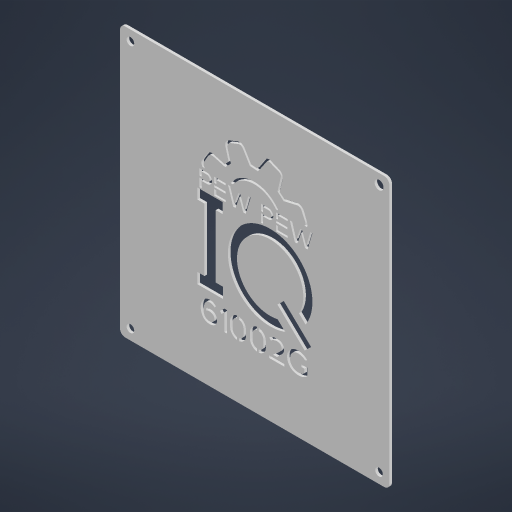
# Autodesk Inventor part: cutout
Saved by Autodesk Inventor 2024 (Build 280153000, 153)
## iProperties
Created: 2023-09-04
Part Number: cutout
Material: Generic
Document SubType Name: Modeling
Designer: reima
Density: 1 g/cm^3
Appearance: Default
Author: reima
Autodesk Inventor part; units mm, degrees
ref_plane "YZ Plane" through (0, 0, 0) normal (1, 0, 0) x (0, 1, 0)
ref_plane "XZ Plane" through (0, 0, 0) normal (0, 1, 0) x (-1, 0, 0)
ref_plane "XY Plane" through (0, 0, 0) normal (0, 0, 1) x (1, 0, 0)
sketch "Sketch1" plane through (0, 0, 0) normal (0, 0, 1) x (1, 0, 0)
  line L0 (-79.375, 82.55) -> (79.375, 82.55)
  line L1 (82.55, 79.375) -> (82.55, -79.375)
  line L2 (79.375, -82.55) -> (-79.375, -82.55)
  line L3 (-82.55, -79.375) -> (-82.55, 79.375)
  arc A0 (-79.375, 82.55) -> (-82.55, 79.375) centre (-79.375, 79.375) ccw
  arc A1 (-82.55, -79.375) -> (-79.375, -82.55) centre (-79.375, -79.375) ccw
  arc A2 (79.375, -82.55) -> (82.55, -79.375) centre (79.375, -79.375) ccw
  arc A3 (82.55, 79.375) -> (79.375, 82.55) centre (79.375, 79.375) ccw
  circle A4 centre (-76.2, 76.2) radius 2.3368
  circle A5 centre (76.2, 76.2) radius 2.7491
  circle A6 centre (76.2, -76.2) radius 2.3368
  circle A7 centre (-76.2, -76.2) radius 2.3368
  point P0 (0, 0)
  point P1 (-82.55, 82.55)
  point P2 (82.55, -82.55)
  point P3 (82.55, 82.55)
  dimension "d0" = 165.1
  dimension "d1" = 165.1
  dimension "d2" = 3.175
  dimension "d3" = 4.6736
  dimension "d4" = 6.35
  dimension "d5" = 6.35
  dimension "d6" = 4.6736
  dimension "d7" = 6.35
  dimension "d8" = 6.35
  dimension "d9" = 6.35
  dimension "d10" = 6.35
  dimension "d11" = 4.6736
  dimension "d12" = 6.35
  dimension "d13" = 6.35
  dimension "d16" = 82.55
  dimension "d17" = 82.55
  constraints: 8 centre point, 8 end point, 8 point on circle, 8 tangent, 6 point on line, 3 equal radius, 2 parallel, 1 horizontal, 1 perpendicular
  measures "d0" distance of point (-82.55, 82.55) point (82.55, 82.55)
  measures "d1" distance of point (82.55, 82.55) point (82.55, -82.55)
  measures "d2" radius of A0
  measures "d3" diameter of A4
  measures "d4" distance from line of L0 A4.centre
  measures "d5" distance from line of L3 A4.centre
  measures "d6" diameter of A7
  measures "d7" distance from line of L3 A7.centre
  measures "d8" distance from line of L2 A7.centre
  measures "d9" distance from line of L0 A5.centre
  measures "d10" distance from line of L1 A5.centre
  measures "d11" diameter of A6
  measures "d12" distance from line of L1 A6.centre
  measures "d13" distance from line of L2 A6.centre
  measures "d16" distance from line of point (0, 0) L0
  measures "d17" distance from line of point (0, 0) L3
extrude "Extrusion1" add sketch "Sketch1" along normal blind 1.5875
sketch "Sketch2" plane through (0, 0, 1.5875) normal (0, 0, 1) x (1, 0, 0)
  line L0 (79.375, 82.55) -> (-79.375, 82.55) projected
  line L1 (-82.55, 79.375) -> (-82.55, -79.375) projected
  line L2 (82.55, -79.375) -> (82.55, 79.375) projected
  line L3 (-79.375, -82.55) -> (79.375, -82.55) projected
  line L4 (-24.8519, 25.6674) -> (-17.8481, 25.6674)
  line L5 (-17.8481, 25.6674) -> (-17.8481, 24.5342)
  line L6 (-17.8481, 24.5342) -> (-24.8519, 24.5342)
  line L7 (-24.8519, 24.5342) -> (-24.8519, 25.6674)
  line L8 (-24.8519, 23.4797) -> (-23.5456, 23.4797)
  line L9 (-23.5456, 23.4797) -> (-23.5456, 20.0486)
  line L10 (-23.5456, 20.0486) -> (-24.8519, 20.0486)
  line L11 (-24.8519, 20.0486) -> (-24.8519, 23.4797)
  line L12 (-23.5456, 20.0486) -> (-17.8481, 20.0486)
  line L13 (-17.8481, 20.0486) -> (-17.8481, 21.1661)
  line L14 (-17.8481, 21.1661) -> (-23.5456, 21.1661)
  line L15 (-23.5456, 21.1661) -> (-23.5456, 20.0486)
  line L16 (-24.8519, 26.8478) -> (-23.5456, 26.8478)
  line L17 (-23.5456, 26.8478) -> (-23.5456, 30.0743)
  line L18 (-23.5456, 30.0743) -> (-24.8519, 30.0743)
  line L19 (-24.8519, 30.0743) -> (-24.8519, 26.8478)
  line L20 (-23.5456, 30.0743) -> (-17.8481, 30.0743)
  line L21 (-17.8481, 30.0743) -> (-17.8481, 28.9568)
  line L22 (-17.8481, 28.9568) -> (-23.5456, 28.9568)
  line L23 (-23.5456, 28.9568) -> (-23.5456, 30.0743)
  line L24 (-33.9115, 26.22) -> (-32.605, 26.22)
  line L25 (-32.605, 26.22) -> (-32.605, 30.0743)
  line L26 (-32.605, 30.0743) -> (-33.9115, 30.0743)
  line L27 (-33.9115, 30.0743) -> (-33.9115, 26.22)
  line L28 (-33.9115, 25.1008) -> (-32.605, 25.1008)
  line L29 (-32.605, 25.1008) -> (-32.605, 20.0486)
  line L30 (-32.605, 20.0486) -> (-33.9115, 20.0486)
  line L31 (-33.9115, 20.0486) -> (-33.9115, 25.1008)
  line L32 (-32.605, 30.0743) -> (-29.4768, 30.0743)
  line L33 (-29.4768, 30.0743) -> (-29.4768, 28.9568)
  line L34 (-29.4768, 28.9568) -> (-32.605, 28.9568)
  line L35 (-32.605, 28.9568) -> (-32.605, 30.0743)
  line L36 (-32.605, 25.1008) -> (-29.4768, 25.1008)
  line L37 (-29.4768, 25.1008) -> (-29.4768, 24.0088)
  line L38 (-29.4768, 24.0088) -> (-32.605, 24.0088)
  line L39 (-32.605, 24.0088) -> (-32.605, 25.1008)
  arc A0 (-29.4768, 25.1008) -> (-29.4768, 28.9568) centre (-29.4768, 27.0288) ccw
  arc A1 (-29.4768, 24.0088) -> (-29.4768, 30.0743) centre (-29.2319, 27.0416) ccw
  line L40 (-16.4079, 30.0743) -> (-15.0487, 30.0064)
  line L41 (-15.0487, 30.0064) -> (-12.5084, 21.995)
  line L42 (-12.5084, 21.995) -> (-9.9795, 28.8267)
  line L43 (-9.9795, 28.8267) -> (-8.8388, 28.8267)
  line L44 (-8.8388, 28.8267) -> (-6.3295, 21.6605)
  line L45 (-6.3295, 21.6605) -> (-3.9885, 30.0743)
  line L46 (-3.9885, 30.0743) -> (-2.5145, 30.0743)
  line L47 (-2.5145, 30.0743) -> (-5.4869, 20.0486)
  line L48 (-5.4869, 20.0486) -> (-7.0427, 20.0486)
  line L49 (-7.0427, 20.0486) -> (-9.4296, 26.8478)
  line L50 (-9.4296, 26.8478) -> (-11.7613, 20.0486)
  line L51 (-11.7613, 20.0486) -> (-13.2289, 20.0486)
  line L52 (-16.4079, 30.0743) -> (-13.2289, 20.0486)
  line L53 (3.7905, 26.22) -> (5.0925, 26.22)
  line L54 (5.0925, 26.22) -> (5.0925, 30.0743)
  line L55 (5.0925, 30.0743) -> (3.7905, 30.0743)
  line L56 (3.7905, 30.0743) -> (3.7905, 26.22)
  line L57 (3.7905, 25.0615) -> (5.0925, 25.0615)
  line L58 (5.0925, 25.0615) -> (5.0925, 20.0486)
  line L59 (5.0925, 20.0486) -> (3.7905, 20.0486)
  line L60 (3.7905, 20.0486) -> (3.7905, 25.0615)
  line L61 (5.0925, 30.0743) -> (8.1235, 30.0743)
  line L62 (8.1235, 30.0743) -> (8.1235, 28.9568)
  line L63 (8.1235, 28.9568) -> (5.0925, 28.9568)
  line L64 (5.0925, 28.9568) -> (5.0925, 30.0743)
  line L65 (5.0925, 25.0615) -> (8.1235, 25.0615)
  line L66 (8.1235, 25.0615) -> (8.1235, 24.0088)
  line L67 (8.1235, 24.0088) -> (5.0925, 24.0088)
  line L68 (5.0925, 24.0088) -> (5.0925, 25.0615)
  arc A2 (8.1235, 25.0615) -> (8.1235, 28.9568) centre (8.2489, 27.0091) ccw
  arc A3 (8.1235, 24.0088) -> (8.1235, 30.0743) centre (8.318, 27.0416) ccw
  line L69 (12.9709, 30.0743) -> (20.1584, 30.0743)
  line L70 (20.1584, 30.0743) -> (20.1584, 28.9568)
  line L71 (20.1584, 28.9568) -> (12.9709, 28.9568)
  line L72 (12.9709, 28.9568) -> (12.9709, 30.0743)
  line L73 (12.9709, 30.0743) -> (14.2728, 30.0743)
  line L74 (14.2728, 30.0743) -> (14.2728, 26.8478)
  line L75 (14.2728, 26.8478) -> (12.9709, 26.8478)
  line L76 (12.9709, 26.8478) -> (12.9709, 30.0743)
  line L77 (12.9709, 25.6674) -> (19.9716, 25.6674)
  line L78 (19.9716, 25.6674) -> (19.9716, 24.5352)
  line L79 (19.9716, 24.5352) -> (12.9709, 24.5352)
  line L80 (12.9709, 24.5352) -> (12.9709, 25.6674)
  line L81 (12.9709, 23.4482) -> (14.2728, 23.4482)
  line L82 (14.2728, 23.4482) -> (14.2728, 20.0486)
  line L83 (14.2728, 20.0486) -> (12.9709, 20.0486)
  line L84 (12.9709, 20.0486) -> (12.9709, 23.4482)
  line L85 (14.2728, 20.0486) -> (20.1584, 20.0486)
  line L86 (20.1584, 20.0486) -> (20.1584, 21.1661)
  line L87 (20.1584, 21.1661) -> (14.2728, 21.1661)
  line L88 (14.2728, 21.1661) -> (14.2728, 20.0486)
  line L89 (21.5158, 30.0743) -> (22.9913, 30.0743)
  line L90 (22.9913, 30.0743) -> (25.3697, 21.9057)
  line L91 (25.3697, 21.9057) -> (27.9414, 28.8267)
  line L92 (27.9414, 28.8267) -> (29.0321, 28.8267)
  line L93 (29.0321, 28.8267) -> (31.5461, 21.6605)
  line L94 (31.5461, 21.6605) -> (34.0406, 30.0743)
  line L95 (34.0406, 30.0743) -> (35.364, 30.0743)
  line L96 (35.364, 30.0743) -> (32.3916, 20.0486)
  line L97 (32.3916, 20.0486) -> (30.821, 20.0486)
  line L98 (30.821, 20.0486) -> (28.4867, 26.9432)
  line L99 (28.4867, 26.9432) -> (26.1223, 20.0486)
  line L100 (26.1223, 20.0486) -> (24.5757, 20.0486)
  line L101 (24.5757, 20.0486) -> (21.5158, 30.0743)
  line L102 (-14.8184, 31.7504) -> (-13.3796, 31.7504)
  line L103 (14.4691, 31.7504) -> (12.9504, 31.7504)
  arc A4 (12.9504, 31.7504) -> (-13.3796, 31.7504) centre (-0.2146, 22.0306) ccw
  arc A5 (14.4691, 31.7504) -> (-14.8184, 31.7504) centre (-0.1747, 22.2165) ccw
  arc A6 (-30.8376, 35.2446) -> (-30.528, 31.7301) centre (-28.5658, 33.6739) ccw
  arc A7 (-24.9796, 40.4718) -> (-28.5658, 39.1347) centre (-25.9768, 37.6683) ccw
  arc A8 (-7.2899, 53.8438) -> (-10.3551, 54.6808) centre (-9.252, 52.6894) ccw
  arc A9 (9.174, 54.763) -> (7.322, 54.1112) centre (8.6906, 53.1796) ccw
  arc A10 (15.9892, 50.348) -> (15.2336, 52.3036) centre (14.2988, 50.8186) ccw
  arc A11 (30.4954, 31.7302) -> (30.6342, 34.6691) centre (28.6879, 33.2883) ccw
  arc A12 (28.7936, 38.6923) -> (26.0478, 40.3102) centre (26.5711, 38.0594) ccw
  line L104 (17.7398, 38.395) -> (26.0478, 40.3102)
  line L105 (28.7936, 38.6923) -> (30.6342, 34.6691)
  line L106 (30.4954, 31.7302) -> (31.9789, 31.7302)
  line L107 (-7.2899, 53.8438) -> (-2.9717, 46.7093)
  line L108 (-2.9717, 46.7093) -> (2.0382, 46.3701)
  line L109 (2.0382, 46.3701) -> (7.322, 54.1112)
  line L110 (9.174, 54.763) -> (15.2336, 52.3036)
  line L111 (15.9892, 50.348) -> (13.9731, 41.6604)
  line L112 (13.9731, 41.6604) -> (17.7398, 38.395)
  line L113 (-30.8376, 35.2446) -> (-28.5658, 39.1347)
  line L114 (-24.9796, 40.4718) -> (-18.0625, 38.5471)
  line L115 (-18.0625, 38.5471) -> (-14.6127, 42.0733)
  line L116 (-14.6127, 42.0733) -> (-16.6084, 49.3312)
  line L117 (-30.528, 31.7301) -> (-32.0036, 31.7301)
  arc A13 (-32.3999, 35.0685) -> (-32.0036, 31.7301) centre (-29.3965, 33.7324) ccw
  arc A14 (-25.3886, 41.886) -> (-27.8196, 41.5513) centre (-26.1227, 38.2222) ccw
  line L118 (-32.3999, 35.0685) -> (-28.8099, 40.8187)
  arc A15 (-27.8196, 41.5513) -> (-28.8099, 40.8187) centre (-26.1228, 38.2221) ccw
  line L119 (-25.3886, 41.886) -> (-18.5094, 39.8807)
  line L120 (-18.5094, 39.8807) -> (-15.9824, 42.4637)
  line L121 (-15.9824, 42.4637) -> (-17.782, 49.0085)
  arc A16 (-15.4658, 52.6898) -> (-16.6084, 49.3312) centre (-13.5626, 50.1687) ccw
  line L122 (-15.4658, 52.6898) -> (-10.3551, 54.6808)
  arc A17 (-16.0392, 53.8438) -> (-17.9814, 49.7337) centre (-14.5412, 50.622) ccw
  line L123 (-17.9814, 49.7337) -> (-17.782, 49.0085)
  arc A18 (-6.1258, 54.5484) -> (-10.1949, 56.0828) centre (-9.119, 52.7734) ccw
  line L124 (-16.0392, 53.8438) -> (-10.1949, 56.0828)
  line L125 (-6.1258, 54.5484) -> (-2.1918, 47.9531)
  line L126 (-2.1918, 47.9531) -> (1.4246, 47.6353)
  arc A19 (10.2006, 55.7927) -> (6.1245, 54.7631) centre (8.8209, 52.6717) ccw
  line L127 (1.4246, 47.6353) -> (6.1245, 54.7631)
  arc A20 (17.0893, 49.5812) -> (15.5262, 53.5334) centre (13.7637, 50.5511) ccw
  line L128 (17.0893, 49.5812) -> (15.3353, 42.0229)
  line L129 (10.2006, 55.7927) -> (15.5262, 53.5334)
  line L130 (15.3353, 42.0229) -> (18.1443, 39.6904)
  arc A21 (30.2891, 39.005) -> (25.8497, 41.5513) centre (26.659, 37.8191) ccw
  line L131 (25.8497, 41.5513) -> (18.1443, 39.6904)
  arc A22 (31.9789, 31.7302) -> (32.1682, 34.1841) centre (29.8071, 33.132) ccw
  line L132 (30.2891, 39.005) -> (32.1682, 34.1841)
  line L133 (-35.213, 19.1945) -> (-19.5698, 19.1945)
  line L134 (-19.5698, 19.1945) -> (-19.5698, 12.8212)
  line L135 (-19.5698, 12.8212) -> (-35.213, 12.8212)
  line L136 (-35.213, 12.8212) -> (-35.213, 19.1945)
  line L137 (-30.7892, 12.8212) -> (-23.8688, 12.8212)
  line L138 (-23.8688, 12.8212) -> (-23.8688, -25.645)
  line L139 (-23.8688, -25.645) -> (-30.7892, -25.645)
  line L140 (-30.7892, -25.645) -> (-30.7892, 12.8212)
  line L141 (-35.213, -25.645) -> (-19.5138, -25.645)
  line L142 (-19.5138, -25.645) -> (-19.5138, -32.1253)
  line L143 (-19.5138, -32.1253) -> (-35.213, -32.1253)
  line L144 (-35.213, -32.1253) -> (-35.213, -25.645)
  line L145 (17.8686, -14.6278) -> (13.8767, -18.395)
  line L146 (13.8767, -18.395) -> (30.6342, -34.4875)
  line L147 (30.6342, -34.4875) -> (34.6261, -30.7203)
  line L148 (34.6261, -30.7203) -> (17.8686, -14.6278)
  arc A23 (27.1093, -16.4401) -> (14.0046, -26.1551) centre (9.4734, -6.3468) ccw
  arc A24 (31.9416, -19.2058) -> (15.2462, -31.5827) centre (9.4734, -6.3468) ccw
  line L149 (14.0046, -26.1551) -> (18.6982, -30.5352)
  arc A25 (15.2462, -31.5827) -> (18.6982, -30.5352) centre (9.4734, -6.3468) ccw
  line L150 (27.1093, -16.4401) -> (31.1956, -20.4294)
  arc A26 (31.1956, -20.4294) -> (31.949, -19.1929) centre (9.4734, -6.3468) ccw
  line L151 (-16.961, -49.284) -> (-18.6004, -49.284)
  line L152 (-18.6004, -49.284) -> (-18.6004, -36.8327)
  line L153 (-18.6004, -36.8327) -> (-16.961, -36.8327)
  line L154 (-16.961, -36.8327) -> (-16.961, -49.284)
  line L155 (-18.6004, -36.8327) -> (-21.35, -39.4034)
  line L156 (-21.35, -39.4034) -> (-20.2834, -40.5442)
  line L157 (-20.2834, -40.5442) -> (-18.6004, -38.8165)
  line L158 (8.8648, -47.9011) -> (18.2227, -47.9011)
  line L159 (18.2227, -47.9011) -> (18.2227, -49.284)
  line L160 (18.2227, -49.284) -> (8.8648, -49.284)
  line L161 (8.8648, -49.284) -> (8.8648, -47.9011)
  line L162 (28.559, -42.8648) -> (32.2489, -42.8648)
  line L163 (32.2489, -42.8648) -> (32.2489, -44.216)
  line L164 (32.2489, -44.216) -> (28.559, -44.216)
  line L165 (28.559, -44.216) -> (28.559, -42.8648)
  line L166 (-24.5421, -39.1949) -> (-23.7981, -38.118)
  arc A27 (-23.7981, -38.118) -> (-32.0782, -39.1949) centre (-27.5277, -41.8118) ccw
  arc A28 (-32.0782, -39.1949) -> (-31.5922, -47.9011) centre (-25.0317, -43.1683) ccw
  arc A29 (-31.5922, -47.9011) -> (-24.8519, -48.7501) centre (-27.7037, -44.2105) ccw
  arc A30 (-24.8519, -48.7501) -> (-23.4202, -43.7641) centre (-27.0708, -45.4145) ccw
  arc A31 (-23.4202, -43.7641) -> (-27.1885, -41.472) centre (-26.7816, -45.0466) ccw
  line L167 (-29.7906, -42.2565) -> (-29.7906, -43.2994)
  arc A32 (-25.7118, -43.4813) -> (-29.7906, -43.2994) centre (-27.9049, -46.8361) ccw
  line L168 (-27.1885, -41.472) -> (-28.3737, -41.472)
  arc A33 (-28.3737, -41.472) -> (-29.7906, -42.2565) centre (-28.4926, -42.9291) ccw
  arc A34 (-25.8864, -47.5561) -> (-25.7118, -43.4813) centre (-27.1461, -45.461) ccw
  arc A35 (-30.703, -46.5882) -> (-25.8864, -47.5561) centre (-27.8144, -44.6818) ccw
  arc A36 (-31.3171, -43.1683) -> (-30.703, -46.5882) centre (-25.48, -43.8852) ccw
  arc A37 (-30.7892, -40.3427) -> (-31.3171, -43.1683) centre (-15.1595, -44.725) ccw
  arc A38 (-26.8428, -38.0151) -> (-30.7892, -40.3427) centre (-27.433, -41.5238) ccw
  arc A39 (-24.5421, -39.1949) -> (-26.8428, -38.0151) centre (-28.5537, -44.1848) ccw
  arc A40 (-6.8639, -41.3097) -> (-13.5626, -41.3297) centre (-10.2129, -41.4212) ccw
  arc A41 (-13.5626, -44.9246) -> (-6.8639, -44.9246) centre (-10.2132, -44.7281) ccw
  line L169 (-13.5626, -41.3297) -> (-13.5626, -44.9246)
  line L170 (-6.8639, -41.3097) -> (-6.8639, -44.9246)
  arc A42 (5.2396, -41.3097) -> (-1.3131, -41.3097) centre (1.9632, -41.346) ccw
  arc A43 (-1.3131, -45.0466) -> (5.2396, -44.9246) centre (1.9597, -44.7941) ccw
  line L171 (-1.3131, -41.3097) -> (-1.3131, -45.0466)
  line L172 (5.2396, -41.3097) -> (5.2396, -44.9246)
  arc A44 (-5.3567, -41.2869) -> (-15.0698, -41.311) centre (-10.2129, -41.4212) ccw
  line L173 (-5.3567, -41.2869) -> (-5.3567, -44.9647)
  arc A45 (-15.0698, -44.9647) -> (-5.3567, -44.9647) centre (-10.2132, -44.7281) ccw
  line L174 (-15.0698, -44.9647) -> (-15.0698, -41.311)
  arc A46 (-2.9246, -45.1025) -> (6.8511, -44.9535) centre (1.9597, -44.7941) ccw
  line L175 (6.8511, -44.9535) -> (6.8511, -41.3016)
  arc A47 (6.8511, -41.3016) -> (-2.9246, -41.3016) centre (1.9632, -41.346) ccw
  line L176 (-2.9246, -41.3016) -> (-2.9246, -45.1025)
  arc A48 (14.4691, -38.0695) -> (9.9205, -39.5089) centre (13.7247, -43.6238) ccw
  arc A49 (16.0784, -38.9953) -> (14.4691, -38.0695) centre (13.7834, -41.1229) ccw
  arc A50 (16.2123, -41.472) -> (16.0784, -38.9953) centre (13.9632, -40.3516) ccw
  arc A51 (13.8767, -44.1033) -> (16.2123, -41.472) centre (8.8032, -37.2477) ccw
  line L177 (11.1363, -46.3974) -> (13.8767, -44.1033)
  line L178 (11.1363, -46.3974) -> (13.6219, -46.3974)
  line L179 (13.6219, -46.3974) -> (16.0784, -44.1033)
  arc A52 (16.0784, -44.1033) -> (17.6164, -42.0514) centre (10.1369, -38.0474) ccw
  arc A53 (17.6164, -42.0514) -> (17.7841, -38.8995) centre (14.3385, -40.2966) ccw
  arc A54 (17.7679, -38.8601) -> (14.911, -36.7775) centre (14.5315, -40.2988) ccw
  line L180 (17.7679, -38.8601) -> (17.7841, -38.8995)
  arc A55 (14.911, -36.7775) -> (11.4325, -36.9516) centre (13.7088, -47.5948) ccw
  arc A56 (11.4325, -36.9516) -> (8.8648, -38.4103) centre (12.8598, -42.4531) ccw
  line L181 (8.8648, -38.4103) -> (9.9205, -39.5089)
  line L182 (-9.5656, -36.6064) -> (-10.8602, -36.6064)
  line L183 (-10.8602, -36.6064) -> (-10.8602, -49.6876)
  line L184 (-10.8602, -49.6876) -> (-9.5656, -49.6876)
  line L185 (-9.5656, -49.6876) -> (-9.5656, -36.6064)
  line L186 (1.4246, -36.4878) -> (2.5019, -36.4878)
  line L187 (2.5019, -36.4878) -> (2.5019, -49.6876)
  line L188 (2.5019, -49.6876) -> (1.4246, -49.6876)
  line L189 (1.4246, -49.6876) -> (1.4246, -36.4878)
  line L190 (32.2489, -44.216) -> (32.2489, -47.3387)
  arc A57 (28.2995, -49.3991) -> (32.2489, -47.3387) centre (27.0457, -42.1802) ccw
  arc A58 (23.7631, -48.9111) -> (28.2995, -49.3991) centre (26.8243, -41.7838) ccw
  arc A59 (20.7613, -46.3266) -> (23.7631, -48.9111) centre (25.464, -43.8999) ccw
  arc A60 (19.8977, -42.832) -> (20.7613, -46.3266) centre (25.247, -43.3641) ccw
  arc A61 (20.1584, -40.8766) -> (19.8977, -42.832) centre (24.572, -42.4601) ccw
  arc A62 (23.0457, -37.4369) -> (20.1584, -40.8766) centre (26.5697, -43.3266) ccw
  arc A63 (27.3783, -36.5109) -> (23.0457, -37.4369) centre (26.5697, -43.3266) ccw
  arc A64 (32.1683, -38.8601) -> (27.3783, -36.5109) centre (26.9845, -43.3717) ccw
  line L191 (32.1683, -38.8601) -> (30.9291, -39.6102)
  arc A65 (30.9291, -39.6102) -> (26.3966, -37.9802) centre (26.6308, -44.4458) ccw
  arc A66 (26.3966, -37.9802) -> (23.7275, -38.9465) centre (26.5644, -42.6131) ccw
  arc A67 (23.8428, -38.8601) -> (21.997, -41.1229) centre (26.2549, -42.712) ccw
  arc A68 (21.997, -41.1229) -> (21.7424, -44.4458) centre (29.5751, -43.3746) ccw
  arc A69 (21.7424, -44.4458) -> (23.9729, -47.3387) centre (26.4867, -43.0943) ccw
  arc A70 (23.9729, -47.3387) -> (27.7442, -47.9595) centre (26.6881, -42.6096) ccw
  arc A71 (27.7442, -47.9595) -> (30.4346, -46.6359) centre (27.5309, -44.1301) ccw
  line L192 (30.4346, -46.6359) -> (30.4346, -44.216)
  point P0 (0, 0)
  point P1 (-72.9862, 2.7952)
  point P2 (0, 72.9862)
  point P3 (0, 82.55)
  point P4 (0, 82.55)
  point P5 (31.9416, -19.2058)
  point P6 (2.5019, -48.0316)
  point P7 (2.5019, -49.658)
  point P8 (2.5019, -38.114)
  point P9 (1.4246, -38.114)
  point P10 (1.4246, -49.6588)
  point P11 (1.4246, -48.0328)
  point P12 (-9.5656, -48.02)
  point P13 (-9.5656, -49.547)
  point P14 (-9.5656, -38.1334)
  point P15 (-10.8602, -38.1334)
  point P16 (-10.8602, -49.5471)
  point P17 (-10.8602, -48.0202)
  point P18 (14.2728, 28.9568)
  dimension "d127" = 20.32
  constraints: 379 end point, 154 point on circle, 72 centre point, 63 parallel, 38 horizontal, 28 point on line, 27 perpendicular, 5 tangent, 5 vertical, 2 concentric, 2 midpoint, 13 other
  measures "d127" radius of A23
extrude "Extrusion2" cut sketch "Sketch2" against normal blind 1.5875 contours L133 L134 L135 L136 | L135 L138 L139 L140 | L139 L141 L142 L143 L144 | L148 L147 L146 L145 | A23 L149 A25 A24 A26 L150 | L151 L152 L153 L154 | L157 L156 L155 L152 | L158 L159 L160 L161 | L162 L163 L164 L165 | L190 A57 A58 A59 A60 A61 A62 A63 A64 L191 A65 A66 A67 A68 A69 A70 A71 L192 L164 | A39 A38 A37 A36 A35 A34 A32 L167 A33 L168 A31 A30 A29 A28 A27 L166 | A40 L185 A44 L173 A45 A41 L170 | A40 L169 A41 L183 A45 L174 A44 | A42 L187 A47 L175 A46 A43 L172 | A42 L171 A43 L189 A46 L176 A47 | A48 L181 A56 A55 A54 L180 A53 A52 L179 L178 L177 A51 A50 A49
extrude "Extrusion3" cut sketch "Sketch2" against normal blind 1.5875 contours L4 L5 L6 L7 | L8 L9 L10 L11 | L14 L13 L12 L9 | L19 L18 L17 L16 | L17 L20 L21 L22 | L27 L26 L25 L24 | L25 L32 L33 L34 | L33 A1 L37 A0 | L37 L38 L29 L36 | L29 L30 L31 L28 | L40 L41 L42 L43 L44 L45 L46 L47 L48 L49 L50 L51 L52 | L56 L55 L54 L53 | L54 L61 L62 L63 | L62 A3 L66 A2 | L66 L67 L58 L65 | L58 L59 L60 L57 | L69 L74 L71 L72 | L69 L70 L71 L74 | L71 L74 L75 L76 | L77 L78 L79 L80 | L81 L82 L83 L84 | L87 L86 L85 L82 | L89 L90 L91 L92 L93 L94 L95 L96 L97 L98 L99 L100 L101 | A5 L103 A4 L102 | A6 L117 A13 L118 A15 A14 L119 L120 L121 L123 A17 L124 A18 L125 L126 L127 A19 L129 A20 L128 L130 L131 A21 L132 A22 L106 A11 L105 A12 L104 L112 L111 A10 L110 A9 L109 L108 L107 A8 L122 A16 L116 L115 L114 A7 L113
body "Solid1"
